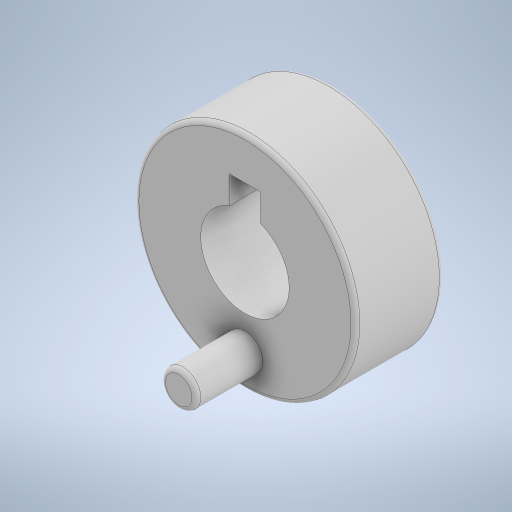
# Autodesk Inventor part: PIEZA PARA GIRAR
Saved by Autodesk Inventor 2024 (Build 280153000, 153)
## iProperties
Created: 2024-03-27
Part Number: PIEZA PARA GIRAR
Material: Genérico
Document SubType Name: Modeling
Designer: kelly
Density: 1 g/cm^3
Appearance: Valor por defecto
Author: kelly
Autodesk Inventor part; units mm, degrees
ref_plane "YZ Plane" through (0, 0, 0) normal (1, 0, 0) x (0, 1, 0)
ref_plane "XZ Plane" through (0, 0, 0) normal (0, 1, 0) x (-1, 0, 0)
ref_plane "XY Plane" through (0, 0, 0) normal (0, 0, 1) x (1, 0, 0)
sketch "Boceto1" plane through (0, 0, 0) normal (0, 0, 1) x (1, 0, 0)
  circle A0 centre (0, 0) radius 25
  circle A1 centre (0, 0) radius 10
  line L0 (0, -25) -> (0, -17.5)
  circle A2 centre (0, -17.5) radius 4
  dimension "d0" = 50
  dimension "d1" = 20
  dimension "d3" = 7.5
  dimension "d4" = 8
  constraints: 3 coincident, 2 centre point, 2 end point, 1 vertical, 1 vertical alignment, 2 other
  measures "d1" diameter of A1
  measures "d3" distance of L0.start L0.end
  measures "d4" diameter of A2
extrude "Extrusión1" add sketch "Boceto1" along normal blind 35 contours A2
extrude "Extrusión2" add sketch "Boceto1" along normal blind 20
fillet "Empalme1" radius 1 3 edges at (-25, 0, 0) (-25, 0, 20) (-4, -17.5, 35)
sketch "Boceto3" plane through (0, 0, 20) normal (0, 0, 1) x (1, 0, 0)
  line L0 (0, 15.6) -> (-3.5, 15.6)
  line L1 (-3.5, 15.6) -> (-3.5, 5.6)
  line L2 (-3.5, 5.6) -> (3.5, 5.6)
  line L3 (3.5, 5.6) -> (3.5, 15.6)
  line L4 (3.5, 15.6) -> (0, 15.6)
  point P0 (0, 0)
  dimension "d18" = 15.6
  dimension "d19" = 3.5
  dimension "d20" = 10
  dimension "d21" = 7
  constraints: 10 end point, 4 perpendicular, 1 point on line
  measures "d18" distance of point (0, 0) L0.start
  measures "d19" distance of L0.start L0.end
  measures "d20" distance of L0.end L1.end
  measures "d21" distance of L1.end L2.end
extrude "Extrusión4" cut sketch "Boceto3" against normal through all
